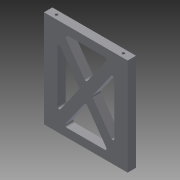
# Autodesk Inventor part: Link_Supporter
Saved by Autodesk Inventor 2013 (Build 170138000, 138)
## iProperties
Created: 2014-05-20
Part Number: Link_Supporter
Material: 一般
Document SubType Name: Modeling
Designer: andou
Density: 1 g/cm^3
Author: andou
Autodesk Inventor part; units mm, degrees
ref_plane "YZ Plane" through (0, 0, 0) normal (1, 0, 0) x (0, 1, 0)
ref_plane "XZ Plane" through (0, 0, 0) normal (0, 1, 0) x (-1, 0, 0)
ref_plane "XY Plane" through (0, 0, 0) normal (0, 0, 1) x (1, 0, 0)
sketch "スケッチ1" plane through (0, 0, 0) normal (0, 0, 1) x (1, 0, 0)
  line L0 (25, 2.5) -> (25, -2.5)
  line L1 (25, -2.5) -> (-25, -2.5)
  line L2 (-25, -2.5) -> (-25, 2.5)
  line L3 (-25, 2.5) -> (25, 2.5)
  point P0 (0, 0)
  dimension "d6" = 50
  dimension "d11" = 2.5
  dimension "d12" = 25
  dimension "d17" = 5
  constraints: 8 end point, 2 parallel, 2 perpendicular
  measures "d6" distance of L0.end L1.end
  measures "d11" distance from line of point (0, 0) L1
  measures "d12" distance from line of point (0, 0) L0
  measures "d17" distance of L1.end L2.end
extrude "押し出し2" add sketch "スケッチ1" along normal blind 58
sketch "スケッチ2" plane through (0, 0, 58) normal (0, 0, 1) x (1, 0, 0)
  line L0 (25, 2.5) -> (-25, 2.5) projected
  circle A0 centre (-20, 0) radius 1
  circle A1 centre (20, 0) radius 1
  point P0 (0, 0)
  dimension "d20" = 2
  dimension "d22" = 40
  dimension "d23" = 20
  dimension "d24" = 2.5
  dimension "d25" = 2.5
  constraints: 2 centre point, 1 equal radius
  measures "d20" diameter of A0
  measures "d22" distance of A1.centre A0.centre
  measures "d23" distance of point (0, 0) A0.centre
  measures "d24" distance from line of L0 A0.centre
  measures "d25" distance from line of L0 A1.centre
hole "穴1" at (-20, 0, 58) at (20, 0, 58) direction (0, 0, -1) diameter 1.6 end through all
sketch "スケッチ3" plane through (-25, 2.5, 0) normal (0, 1, 0) x (1, 0, 0)
  line L0 (50, 0) -> (0, 0) projected
  line L1 (0, 0) -> (0, -58) projected
  line L2 (50, -58) -> (0, -58) projected
  line L3 (50, 0) -> (50, -58) projected
  line L4 (8, -5) -> (8, -53)
  line L5 (8, -53) -> (42, -5)
  line L6 (42, -5) -> (42, -53)
  line L7 (42, -53) -> (8, -5)
  line L8 (8, -5) -> (42, -5)
  line L9 (42, -53) -> (8, -53)
  line L10 (8, -10.1902) -> (38.3236, -53)
  line L11 (42, -47.8098) -> (11.6764, -5)
  line L12 (38.3236, -5) -> (8, -47.8098)
  line L13 (11.6764, -53) -> (42, -10.1902)
  point P0 (25, 0)
  dimension "d35" = 5
  dimension "d36" = 5
  dimension "d37" = 8
  dimension "d38" = 8
  dimension "d39" = 6
  dimension "d40" = 6
  constraints: 20 end point, 9 parallel, 8 point on line, 1 perpendicular
  measures "d35" distance between parallel lines of L0 L8
  measures "d36" distance between parallel lines of L9 L2
  measures "d37" distance between parallel lines of L1 L4
  measures "d38" distance between parallel lines of L3 L6
  measures "d39" distance between parallel lines of L13 L12
  measures "d40" distance between parallel lines of L11 L10
extrude "押し出し3" cut sketch "スケッチ3" against normal blind 5 contours L3 L2 L1 L0 | L7 L12 L10 L4 | L8 L11 L12 L7 | L12 L11 L5 L7 | L7 L5 L10 L12 | L12 L10 L5 L4 | L7 L13 L10 L5 | L5 L11 L13 L7 | L12 L8 L5 L11 | L5 L10 L13 L9 | L5 L6 L13 L11 | L13 L11 L6 L7 | L7 L9 L10 L13 keep common part
fillet "フィレット1" radius 1 12 edges at (-13.3236, 0, 5) (-17, 0, 10.1902) (0, 0, 23.8098) (-17, 0, 47.8098) (-3.6764, 0, 29) (13.3236, 0, 5) (0, 0, 34.1902) (17, 0, 10.1902) (17, 0, 47.8098) (13.3236, 0, 53) (-13.3236, 0, 53) (3.6764, 0, 29)
